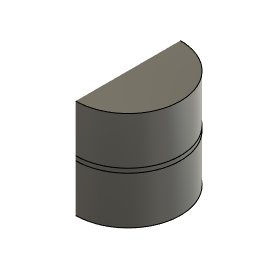
Mill case (Autodesk Fusion 360 design; units mm, degrees)
Autodesk Fusion 360 part; units mm, degrees
note: some values were not read from the file. Set by a fixed rule: which face or edge a step refers to.
sketch "Sketch1" plane through (0, 0, 0) normal (0, 1, 0) x (1, 0, 0)
  circle A0 centre (0, 0) radius 33.5
  circle A1 centre (0, 0) radius 36.5
  dimension "d3" = 67
  dimension "d4" = 73
  constraint coincident A0.centre A1.centre
  constraint concentric A0 A1
  measures "d3" diameter of A0
  measures "d4" diameter of A1
extrude "Extrude1" add sketch "Sketch1" along normal blind 30 makes body 1
extrude "Extrude2" add sketch "Sketch1" against normal blind 3 contours A0 | A1 bodies 1
sketch "Sketch2" plane through (0, -3, 0) normal (0, -1, 0) x (1, 0, 0)
  circle A0 centre (0, 0) radius 36.5
  circle A1 centre (0, 0) radius 36.5
  circle A2 centre (0, 0) radius 33
  circle A3 centre (0, 0) radius 12.5
  line L0 (0, 0) -> (25, 0)
  circle A4 centre (25, 0) radius 1
  circle A5 centre (0, 25) radius 1
  circle A6 centre (-25, 0) radius 1
  circle A7 centre (0, -25) radius 1
  line L1 (0, 0) -> (9.5671, 23.097)
  line L2 (0, 0) -> (25, 0) construction
  line L3 (9.5671, 23.097) -> (10.7151, 25.8686)
  line L4 (10.7151, 25.8686) -> (15.5655, 23.8595)
  line L5 (15.5655, 23.8595) -> (13.2694, 18.3163)
  line L6 (13.2694, 18.3163) -> (3.5687, 22.3344)
  line L7 (3.5687, 22.3344) -> (5.8648, 27.8777)
  line L8 (5.8648, 27.8777) -> (10.7151, 25.8686)
  circle A8 centre (-25, 0) radius 1.5
  circle A9 centre (0, 25) radius 1.5
  circle A10 centre (25, 0) radius 1.5
  circle A11 centre (0, -25) radius 1
  circle A12 centre (0, -25) radius 1.5
  dimension "d12" = 25
  dimension "d13" = 25
  dimension "d14" = 2
  dimension "d16" = 360
  dimension "d19" = 25
  dimension "d20" = 67.5
  dimension "d21" = 3
  dimension "d22" = 5.25
  dimension "d23" = 6
  dimension "d24" = 10.5
  dimension "d29" = 3
  dimension "d30" = 3
  dimension "d31" = 3
  dimension "d32" = 2
  dimension "d33" = 3
  dimension "d36" = 66
  constraint concentric A0 A1
  constraint concentric A0 A2
  constraint concentric A1 A3
  constraint coincident A0.centre A1.centre
  constraint horizontal L0
  constraint coincident L0.end A4.centre
  constraint horizontal L2
  constraint parallel L1 L3
  constraint perpendicular L3 L4
  constraint perpendicular L4 L5
  constraint perpendicular L1 L6
  constraint perpendicular L4 L7
  constraint perpendicular L3 L8
  constraint concentric A6 A8
  constraint concentric A5 A9
  constraint concentric A7 A11
  constraint concentric A11 A12
  measures "d12" diameter of A3
  measures "d13" distance of A0.centre L0.end
  measures "d14" diameter of A4
  measures "d19" distance of A0.centre L1.end
  measures "d20" angle of L1 L2
  measures "d21" distance of L1.end L3.end
  measures "d22" distance of L3.end L4.end
  measures "d23" distance of L4.end L5.end
  measures "d24" distance of L5.end L6.end
  measures "d29" diameter of A8
  measures "d30" diameter of A9
  measures "d31" diameter of A10
  measures "d32" diameter of A11
  measures "d33" diameter of A12
  measures "d36" diameter of A2
extrude "Extrude5" cut sketch "Sketch2" against normal blind 9 contours L1 L3 L6 L7 L8 | L1 L3 L4 L5 L6 bodies 1
extrude "Extrude4" cut sketch "Sketch2" against normal blind 22 contours A4 | A5 | A6 | A7 A11 bodies 1
extrude "Extrude3" add sketch "Sketch2" along normal blind 30 contours A0 A1 bodies 1
extrude "Extrude6" cut sketch "Sketch2" along normal blind 11 contours A8 | A9 | A10 | A12 bodies 1
sketch "Sketch3" plane through (0, 30, 0) normal (0, 1, 0) x (-1, 0, 0)
  circle A0 centre (0, 0) radius 33.5
  circle A1 centre (0, 0) radius 36.5
  circle A2 centre (0, 0) radius 35.5
  dimension "d57" = 71
  constraint coincident A0.centre A1.centre
  measures "d57" diameter of A2
extrude "Extrude7" add sketch "Sketch3" along normal blind 3 contours A0 | A1 | A2 bodies 1
ref_plane "WorkPlane1" through (0, 0, 0) normal (0, 1, 0) x (1, 0, 0)
split "Split1" by plane through (0, 0, 0) normal (0, 1, 0) bodies 1 makes body 2 at (36.3186, 20, 3.6342)
sketch "Sketch4" plane through (0, 0, 0) normal (0, 1, 0) x (1, 0, 0)
  circle A0 centre (0, 0) radius 33.5
  circle A1 centre (0, 0) radius 30
  dimension "d40" = 60
  constraint coincident A0.centre A1.centre
  constraint concentric A0 A1
  measures "d40" diameter of A1
extrude "Extrude8" add sketch "Sketch4" along normal blind 5 bodies 1
ref_plane "WorkPlane2" through (0, -3, 0) normal (0, -1, 0) x (-1, 0, 0)
split "Split2" by plane through (0, -3, 0) normal (0, -1, 0) bodies 1 makes body 3 at (36.3186, -23, -3.6342)
sketch "Sketch5" plane through (0, -3, 0) normal (0, -1, 0) x (1, 0, 0)
  circle A0 centre (0, 0) radius 33
  circle A1 centre (0, 0) radius 30
  dimension "d44" = 60
  constraint coincident A0.centre A1.centre
  measures "d44" diameter of A1
extrude "Extrude9" add sketch "Sketch5" along normal blind 5 bodies 1
thread "Thread1" "ISO Metric profile 68.0 M68x2 6g" major diameter 67.822 minor diameter 65.5239 pitch 2 angle 60 modelled right hand crest width 0.2789 on face at (33.4584, 3.3333, 1.6698) crest through (33.911, -0.5, 0) on bodies 1
thread "Thread2" "ISO Metric profile 68.0 M68x2 6g" major diameter 67.822 minor diameter 65.5239 pitch 2 angle 60 modelled right hand crest width 0.2789 on face at (32.959, -4.6667, 1.6449) crest through (33.911, -2.5, 0) on bodies 1
ref_plane "WorkPlane3" through (0, 7, 0) normal (0, -1, 0) x (0, 0, -1)
split_face "SplitFace1" 1 faces at (-33.4584, 10, 1.6698) by plane through (0, 7, 0) normal (0, -1, 0) on bodies 2
thread "Thread3" "ISO Metric profile 68.0 M68x2 6H" major diameter 68.2623 minor diameter 66.0224 pitch 2 angle 60 modelled right hand crest width 0.5401 on face at (33.3335, 4.6667, -3.3355) crest through (33.0112, 0.5, 0) on bodies 2
ref_plane "WorkPlane4" through (0, -10, 0) normal (0, 1, 0) x (0, 0, 1)
split_face "SplitFace2" 1 faces at (-32.836, -13, 3.2857) by plane through (0, -10, 0) normal (0, 1, 0) on bodies 3
thread "Thread4" "ISO Metric profile 68.0 M68x2 6H" major diameter 68.2623 minor diameter 66.0224 pitch 2 angle 60 modelled right hand crest width 0.5401 on face at (32.836, -7.6667, 3.2857) crest through (33.0112, -3.5, 0) on bodies 3
sketch "Sketch6" plane through (0, -33, 0) normal (0, -1, 0) x (1, 0, 0)
  circle A0 centre (0, 0) radius 33
  circle A1 centre (0, 0) radius 36.5
extrude "Extrude10" add sketch "Sketch6" along normal blind 3 contours A0 | A1 bodies 3
ref_plane "WorkPlane5" through (0, -14.7, 0) normal (0, -1, 0) x (-1, 0, 0)
sketch "Sketch7" plane through (0, -14.7, 0) normal (0, -1, 0) x (1, 0, 0)
  circle A0 centre (0, 0) radius 36.5
  line L0 (0, 0) -> (-25.8094, -25.8094)
  line L1 (0, 0) -> (-36.5, 0) construction
  line L2 (0, 0) -> (-25.8094, 25.8094)
  point P0 (-25.8094, -25.8094)
  point P1 (-25.8094, 25.8094)
  dimension "d52" = 73
  dimension "d53" = 45
  constraint coincident A0.centre L0.start
  constraint horizontal L1
  constraint coincident A0 P0
  constraint coincident P0 L0.end
  constraint coincident A0 P1
  constraint perpendicular L0 L2
  constraint coincident P1 L2.end
  measures "d52" diameter of A0
  measures "d53" angle of L0 L1
ref_plane "WorkPlane6" through (-25.8094, -14.7, -25.8094) normal (-0.707107, 0, -0.707107) x (0, -1, 0)
sketch "Sketch8" plane through (-25.8094, -14.7, -25.8094) normal (-0.707107, 0, -0.707107) x (0, -1, 0)
hole "Hole1" at (-25.8094, -14.7, -25.8094) direction (0.707107, 0, 0.707107) diameter 10 depth 12 tip angle 118 bodies 3
equation "d20 = 45 deg + 22.5 deg"
equation "d40 = 66.000 mm - 6 mm"
equation "d44 = 66.000 mm - 6 mm"
equation "d51 = 5.1 mm + 1.6 mm + 5 mm"
equation "d57 = 67.000 mm + 4 mm"
